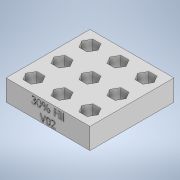
# Autodesk Inventor part: FootPad
Saved by Autodesk Inventor 2021.1 (Build 251245010, 245A)
## iProperties
Created: 2020-09-27
Part Number: FootPad
Material: Generic
Document SubType Name: Modeling
Designer: robst
Density: 1 g/cm^3
Appearance: Default
Author: robst
Autodesk Inventor part; units mm, degrees
ref_plane "YZ Plane" through (0, 0, 0) normal (1, 0, 0) x (0, 1, 0)
ref_plane "XZ Plane" through (0, 0, 0) normal (0, 1, 0) x (-1, 0, 0)
ref_plane "XY Plane" through (0, 0, 0) normal (0, 0, 1) x (1, 0, 0)
sketch "Sketch1" plane through (0, 0, 0) normal (0, 1, 0) x (-1, 0, 0)
  line L0 (-38.1, 38.1) -> (-38.1, -38.1)
  line L1 (-38.1, -38.1) -> (38.1, -38.1)
  line L2 (38.1, -38.1) -> (38.1, 38.1)
  line L3 (38.1, 38.1) -> (-38.1, 38.1)
  line L4 (-38.1, 38.1) -> (38.1, -38.1) construction
  line L5 (-38.1, -38.1) -> (38.1, 38.1) construction
  point P0 (0, 0)
  dimension "d0" = 76.2
  constraints: 12 end point, 2 midpoint, 2 parallel, 2 perpendicular, 1 vertical
  measures "d0" distance of L0.end L1.end
extrude "Extrusion1" add sketch "Sketch1" against normal blind 19.05
sketch "Sketch3" plane through (-38.1, 0, 38.1) normal (0, 0, 1) x (1, 0, 0)
  line L0 (0, 0) -> (0, -19.05) construction
  line L1 (0, -9.525) -> (76.2, -9.525) construction
  line L2 (76.2, 0) -> (76.2, -19.05) construction
  spline S0 degree 2 poles (25.1522, -2.483) (24.9299, -2.483) (24.4902, -2.5917) (24.2778, -2.6756) knots 0 0 0 1 2 2 2
  spline S1 degree 2 poles (24.2778, -2.6756) (24.0802, -2.7596) (23.7887, -2.9375) (23.6751, -3.0165) knots 0 0 0 1 2 2 2
  line L3 (23.6751, -3.0165) -> (23.6257, -3.0165)
  line L4 (23.6257, -3.0165) -> (23.6257, -2.152)
  spline S2 degree 2 poles (23.6257, -2.152) (23.8925, -2.0087) (24.8064, -1.7766) (25.2164, -1.7766) knots 0 0 0 1 2 2 2
  spline S3 degree 2 poles (25.2164, -1.7766) (25.6314, -1.7766) (26.2489, -1.9445) (26.5008, -2.1224) knots 0 0 0 1 2 2 2
  spline S4 degree 2 poles (26.5008, -2.1224) (26.7676, -2.315) (27.0442, -2.8732) (27.0442, -3.2487) knots 0 0 0 1 2 2 2
  spline S5 degree 2 poles (27.0442, -3.2487) (27.0442, -3.7526) (26.3822, -4.5133) (25.9179, -4.6121) knots 0 0 0 1 2 2 2
  line L5 (25.9179, -4.6121) -> (25.9179, -4.6714)
  spline S6 degree 2 poles (25.9179, -4.6714) (26.1105, -4.7109) (26.5502, -4.8888) (26.7379, -5.0666) knots 0 0 0 1 2 2 2
  spline S7 degree 2 poles (26.7379, -5.0666) (26.9256, -5.2395) (27.1628, -5.7928) (27.1628, -6.1929) knots 0 0 0 1 2 2 2
  spline S8 degree 2 poles (27.1628, -6.1929) (27.1628, -6.603) (26.8812, -7.2995) (26.6243, -7.5663) knots 0 0 0 1 2 2 2
  spline S9 degree 2 poles (26.6243, -7.5663) (26.3575, -7.8429) (25.6017, -8.1294) (25.1225, -8.1294) knots 0 0 0 1 2 2 2
  spline S10 degree 2 poles (25.1225, -8.1294) (24.6631, -8.1294) (23.764, -7.9071) (23.4577, -7.754) knots 0 0 0 1 2 2 2
  line L6 (23.4577, -7.754) -> (23.4577, -6.8895)
  line L7 (23.4577, -6.8895) -> (23.517, -6.8895)
  spline S11 degree 2 poles (23.517, -6.8895) (23.7739, -7.0772) (24.6434, -7.423) (25.0731, -7.423) knots 0 0 0 1 2 2 2
  spline S12 degree 2 poles (25.0731, -7.423) (25.3251, -7.423) (25.829, -7.2649) (25.9969, -7.0822) knots 0 0 0 1 2 2 2
  spline S13 degree 2 poles (25.9969, -7.0822) (26.1599, -6.8994) (26.3328, -6.4646) (26.3328, -6.1337) knots 0 0 0 1 2 2 2
  spline S14 degree 2 poles (26.3328, -6.1337) (26.3328, -5.8027) (26.1402, -5.3729) (25.9673, -5.2494) knots 0 0 0 1 2 2 2
  spline S15 degree 2 poles (25.9673, -5.2494) (25.7944, -5.1259) (25.3251, -5.032) (25.0484, -5.032) knots 0 0 0 1 2 2 2
  line L8 (25.0484, -5.032) -> (24.7026, -5.032)
  line L9 (24.7026, -5.032) -> (24.7026, -4.3553)
  line L10 (24.7026, -4.3553) -> (24.9743, -4.3553)
  spline S16 degree 2 poles (24.9743, -4.3553) (25.5227, -4.3553) (26.2143, -3.8316) (26.2143, -3.3327) knots 0 0 0 1 2 2 2
  spline S17 degree 2 poles (26.2143, -3.3327) (26.2143, -3.1005) (26.0364, -2.7695) (25.8932, -2.6707) knots 0 0 0 1 2 2 2
  spline S18 degree 2 poles (25.8932, -2.6707) (25.74, -2.567) (25.3646, -2.483) (25.1522, -2.483) knots 0 0 0 1 2 2 2
  spline S19 degree 2 poles (31.8756, -4.953) (31.8756, -6.5931) (30.9221, -8.1294) (29.9292, -8.1294) knots 0 0 0 1 2 2 2
  spline S20 degree 2 poles (29.9292, -8.1294) (28.9214, -8.1294) (27.9779, -6.5635) (27.9779, -4.9579) knots 0 0 0 1 2 2 2
  spline S21 degree 2 poles (27.9779, -4.9579) (27.9779, -3.308) (28.9313, -1.7815) (29.9292, -1.7815) knots 0 0 0 1 2 2 2
  spline S22 degree 2 poles (29.9292, -1.7815) (30.932, -1.7815) (31.8756, -3.3623) (31.8756, -4.953) knots 0 0 0 1 2 2 2
  spline S23 degree 2 poles (30.8283, -6.8105) (30.9468, -6.5091) (31.0456, -5.5804) (31.0456, -4.953) knots 0 0 0 1 2 2 2
  spline S24 degree 2 poles (31.0456, -4.953) (31.0456, -4.3256) (30.9468, -3.4018) (30.8233, -3.0906) knots 0 0 0 1 2 2 2
  spline S25 degree 2 poles (30.8233, -3.0906) (30.6998, -2.7794) (30.27, -2.4583) (29.9292, -2.4583) knots 0 0 0 1 2 2 2
  spline S26 degree 2 poles (29.9292, -2.4583) (29.5883, -2.4583) (29.1487, -2.7794) (29.0202, -3.1005) knots 0 0 0 1 2 2 2
  spline S27 degree 2 poles (29.0202, -3.1005) (28.8967, -3.4117) (28.8078, -4.3602) (28.8078, -4.9579) knots 0 0 0 1 2 2 2
  spline S28 degree 2 poles (28.8078, -4.9579) (28.8078, -5.6001) (28.8868, -6.4597) (29.0153, -6.7956) knots 0 0 0 1 2 2 2
  spline S29 degree 2 poles (29.0153, -6.7956) (29.1338, -7.1118) (29.5735, -7.4527) (29.9292, -7.4527) knots 0 0 0 1 2 2 2
  spline S30 degree 2 poles (29.9292, -7.4527) (30.2651, -7.4527) (30.7048, -7.1316) (30.8283, -6.8105) knots 0 0 0 1 2 2 2
  spline S31 degree 2 poles (39.9772, -6.3115) (39.9772, -7.2304) (39.2362, -8.1196) (38.5347, -8.1196) knots 0 0 0 1 2 2 2
  spline S32 degree 2 poles (38.5347, -8.1196) (37.8234, -8.1196) (37.0922, -7.2205) (37.0922, -6.3115) knots 0 0 0 1 2 2 2
  spline S33 degree 2 poles (37.0922, -6.3115) (37.0922, -5.3976) (37.8382, -4.5035) (38.5347, -4.5035) knots 0 0 0 1 2 2 2
  spline S34 degree 2 poles (38.5347, -4.5035) (39.251, -4.5035) (39.9772, -5.4025) (39.9772, -6.3115) knots 0 0 0 1 2 2 2
  spline S35 degree 2 poles (35.5164, -3.5994) (35.5164, -4.5183) (34.7754, -5.4075) (34.0739, -5.4075) knots 0 0 0 1 2 2 2
  spline S36 degree 2 poles (34.0739, -5.4075) (33.3625, -5.4075) (32.6314, -4.5084) (32.6314, -3.5994) knots 0 0 0 1 2 2 2
  spline S37 degree 2 poles (32.6314, -3.5994) (32.6314, -2.6855) (33.3773, -1.7914) (34.0739, -1.7914) knots 0 0 0 1 2 2 2
  spline S38 degree 2 poles (34.0739, -1.7914) (34.7902, -1.7914) (35.5164, -2.6905) (35.5164, -3.5994) knots 0 0 0 1 2 2 2
  line L11 (38.2433, -1.905) -> (35.052, -8.001)
  line L12 (35.052, -8.001) -> (34.3752, -8.001)
  line L13 (34.3752, -8.001) -> (37.5665, -1.905)
  line L14 (37.5665, -1.905) -> (38.2433, -1.905)
  spline S39 degree 2 poles (39.251, -6.3115) (39.251, -5.6841) (38.9596, -5.0469) (38.5397, -5.0469) knots 0 0 0 1 2 2 2
  spline S40 degree 2 poles (38.5397, -5.0469) (38.1198, -5.0469) (37.8234, -5.694) (37.8234, -6.3115) knots 0 0 0 1 2 2 2
  spline S41 degree 2 poles (37.8234, -6.3115) (37.8234, -6.929) (38.1, -7.5762) (38.5397, -7.5762) knots 0 0 0 1 2 2 2
  spline S42 degree 2 poles (38.5397, -7.5762) (38.9596, -7.5762) (39.251, -6.929) (39.251, -6.3115) knots 0 0 0 1 2 2 2
  spline S43 degree 2 poles (34.7902, -3.5994) (34.7902, -2.972) (34.4987, -2.3348) (34.0788, -2.3348) knots 0 0 0 1 2 2 2
  spline S44 degree 2 poles (34.0788, -2.3348) (33.6589, -2.3348) (33.3625, -2.9819) (33.3625, -3.5994) knots 0 0 0 1 2 2 2
  spline S45 degree 2 poles (33.3625, -3.5994) (33.3625, -4.2169) (33.6392, -4.8641) (34.0788, -4.8641) knots 0 0 0 1 2 2 2
  spline S46 degree 2 poles (34.0788, -4.8641) (34.4987, -4.8641) (34.7902, -4.2169) (34.7902, -3.5994) knots 0 0 0 1 2 2 2
  line L15 (47.2786, -2.6262) -> (44.443, -2.6262)
  line L16 (44.443, -2.6262) -> (44.443, -4.3454)
  line L17 (44.443, -4.3454) -> (47.16, -4.3454)
  line L18 (47.16, -4.3454) -> (47.16, -5.0666)
  line L19 (47.16, -5.0666) -> (44.443, -5.0666)
  line L20 (44.443, -5.0666) -> (44.443, -8.001)
  line L21 (44.443, -8.001) -> (43.6328, -8.001)
  line L22 (43.6328, -8.001) -> (43.6328, -1.905)
  line L23 (43.6328, -1.905) -> (47.2786, -1.905)
  line L24 (47.2786, -1.905) -> (47.2786, -2.6262)
  line L25 (48.7309, -8.001) -> (47.9603, -8.001)
  line L26 (47.9603, -8.001) -> (47.9603, -3.4265)
  line L27 (47.9603, -3.4265) -> (48.7309, -3.4265)
  line L28 (48.7309, -3.4265) -> (48.7309, -8.001)
  line L29 (48.7853, -2.6658) -> (47.9109, -2.6658)
  line L30 (47.9109, -2.6658) -> (47.9109, -1.8655)
  line L31 (47.9109, -1.8655) -> (48.7853, -1.8655)
  line L32 (48.7853, -1.8655) -> (48.7853, -2.6658)
  line L33 (50.6477, -8.001) -> (49.877, -8.001)
  line L34 (49.877, -8.001) -> (49.877, -1.6333)
  line L35 (49.877, -1.6333) -> (50.6477, -1.6333)
  line L36 (50.6477, -1.6333) -> (50.6477, -8.001)
  line L37 (52.5644, -8.001) -> (51.7938, -8.001)
  line L38 (51.7938, -8.001) -> (51.7938, -1.6333)
  line L39 (51.7938, -1.6333) -> (52.5644, -1.6333)
  line L40 (52.5644, -1.6333) -> (52.5644, -8.001)
  line L41 (36.0622, -11.9717) -> (33.9627, -18.0677)
  line L42 (33.9627, -18.0677) -> (33.0883, -18.0677)
  line L43 (33.0883, -18.0677) -> (30.9888, -11.9717)
  line L44 (30.9888, -11.9717) -> (31.8583, -11.9717)
  line L45 (31.8583, -11.9717) -> (33.5478, -17.0352)
  line L46 (33.5478, -17.0352) -> (35.2373, -11.9717)
  line L47 (35.2373, -11.9717) -> (36.0622, -11.9717)
  spline S47 degree 2 poles (40.3354, -15.0197) (40.3354, -16.6598) (39.3819, -18.1961) (38.389, -18.1961) knots 0 0 0 1 2 2 2
  spline S48 degree 2 poles (38.389, -18.1961) (37.3812, -18.1961) (36.4377, -16.6301) (36.4377, -15.0246) knots 0 0 0 1 2 2 2
  spline S49 degree 2 poles (36.4377, -15.0246) (36.4377, -13.3747) (37.3911, -11.8482) (38.389, -11.8482) knots 0 0 0 1 2 2 2
  spline S50 degree 2 poles (38.389, -11.8482) (39.3918, -11.8482) (40.3354, -13.429) (40.3354, -15.0197) knots 0 0 0 1 2 2 2
  spline S51 degree 2 poles (39.2881, -16.8771) (39.4066, -16.5758) (39.5054, -15.6471) (39.5054, -15.0197) knots 0 0 0 1 2 2 2
  spline S52 degree 2 poles (39.5054, -15.0197) (39.5054, -14.3923) (39.4066, -13.4685) (39.2831, -13.1573) knots 0 0 0 1 2 2 2
  spline S53 degree 2 poles (39.2831, -13.1573) (39.1596, -12.8461) (38.7299, -12.525) (38.389, -12.525) knots 0 0 0 1 2 2 2
  spline S54 degree 2 poles (38.389, -12.525) (38.0481, -12.525) (37.6085, -12.8461) (37.48, -13.1672) knots 0 0 0 1 2 2 2
  spline S55 degree 2 poles (37.48, -13.1672) (37.3565, -13.4784) (37.2676, -14.4269) (37.2676, -15.0246) knots 0 0 0 1 2 2 2
  spline S56 degree 2 poles (37.2676, -15.0246) (37.2676, -15.6668) (37.3466, -16.5264) (37.4751, -16.8623) knots 0 0 0 1 2 2 2
  spline S57 degree 2 poles (37.4751, -16.8623) (37.5936, -17.1785) (38.0333, -17.5193) (38.389, -17.5193) knots 0 0 0 1 2 2 2
  spline S58 degree 2 poles (38.389, -17.5193) (38.7249, -17.5193) (39.1646, -17.1982) (39.2881, -16.8771) knots 0 0 0 1 2 2 2
  line L48 (44.8753, -18.0677) -> (41.1159, -18.0677)
  line L49 (41.1159, -18.0677) -> (41.1159, -17.2032)
  spline S59 degree 2 poles (41.1159, -17.2032) (41.521, -16.8228) (42.2422, -16.1164) (42.588, -15.736) knots 0 0 0 1 2 2 2
  spline S60 degree 2 poles (42.588, -15.736) (43.2846, -14.9703) (43.7934, -14.0514) (43.7934, -13.5624) knots 0 0 0 1 2 2 2
  spline S61 degree 2 poles (43.7934, -13.5624) (43.7934, -13.3055) (43.6353, -12.9202) (43.492, -12.7967) knots 0 0 0 1 2 2 2
  spline S62 degree 2 poles (43.492, -12.7967) (43.3488, -12.6732) (42.9733, -12.5497) (42.7461, -12.5497) knots 0 0 0 1 2 2 2
  spline S63 degree 2 poles (42.7461, -12.5497) (42.5287, -12.5497) (42.0841, -12.6584) (41.8816, -12.7423) knots 0 0 0 1 2 2 2
  spline S64 degree 2 poles (41.8816, -12.7423) (41.7087, -12.8115) (41.3876, -13.0091) (41.2888, -13.0783) knots 0 0 0 1 2 2 2
  line L50 (41.2888, -13.0783) -> (41.2443, -13.0783)
  line L51 (41.2443, -13.0783) -> (41.2443, -12.2088)
  spline S65 degree 2 poles (41.2443, -12.2088) (41.4963, -12.0853) (42.4003, -11.8432) (42.8054, -11.8432) knots 0 0 0 1 2 2 2
  spline S66 degree 2 poles (42.8054, -11.8432) (43.66, -11.8432) (44.6233, -12.7473) (44.6233, -13.5179) knots 0 0 0 1 2 2 2
  spline S67 degree 2 poles (44.6233, -13.5179) (44.6233, -13.8785) (44.4554, -14.4812) (44.3072, -14.7381) knots 0 0 0 1 2 2 2
  spline S68 degree 2 poles (44.3072, -14.7381) (44.1589, -15.0049) (43.7292, -15.5285) (43.492, -15.7805) knots 0 0 0 1 2 2 2
  spline S69 degree 2 poles (43.492, -15.7805) (43.1067, -16.2004) (42.1632, -17.0994) (41.8816, -17.3613) knots 0 0 0 1 2 2 2
  line L52 (41.8816, -17.3613) -> (44.8753, -17.3613)
  line L53 (44.8753, -17.3613) -> (44.8753, -18.0677)
  point P0 (38.1, 0)
  constraints: 2 end point, 2 midpoint, 1 horizontal
extrude "Extrusion3" cut sketch "Sketch3" against normal blind 1.27
sketch "Sketch2" plane through (0, 0, 0) normal (0, 1, 0) x (1, 0, 0)
  line L0 (-38.1, -38.1) -> (38.1, -38.1) projected
  line L1 (38.1, -38.1) -> (38.1, 38.1) projected
  line L2 (29.0662, -19.05) -> (32.7323, -25.4)
  line L3 (32.7323, -25.4) -> (29.0662, -31.75)
  line L4 (29.0662, -31.75) -> (21.7338, -31.75)
  line L5 (21.7338, -31.75) -> (18.0677, -25.4)
  line L6 (18.0677, -25.4) -> (21.7338, -19.05)
  line L7 (21.7338, -19.05) -> (29.0662, -19.05)
  line L8 (38.1, 38.1) -> (-38.1, 38.1) projected
  point P0 (0, 0)
  point P1 (25.4, -25.4)
  dimension "d16" = 12.7
  dimension "d17" = 12.7
  dimension "d18" = 12.7
  constraints: 12 end point, 1 parallel, 13 other
  measures "d16" distance between parallel lines of L4 L7
  measures "d17" distance from line of L0 point (25.4, -25.4)
  measures "d18" distance from line of L1 point (25.4, -25.4)
extrude "Extrusion2" cut sketch "Sketch2" against normal through all
pattern_linear "Rectangular Pattern1" count 3 spacing 25.4 along (-1, 0, 0) count 3 spacing 25.4 along (0, 0, -1) of "Extrusion2"
equation "\"d0\" = width"
equation "\"d1\" = height"
equation "\"width\" = 76.2"
equation "\"height\" = 19.05"
equation "\"holeDiameter\" = 12.7"
body "Solid1"
